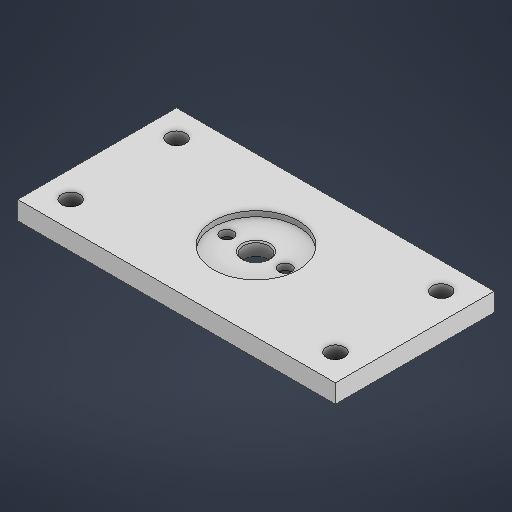
# Autodesk Inventor part: motor mount plate
Saved by Autodesk Inventor 2025.2 (Build 292293000, 293)
## iProperties
Created: 2025-05-10
Part Number: motor mount plate
Material: Generic
Document SubType Name: Modeling
Designer: klawy
Density: 1 g/cm^3
Appearance: Default
Author: klawy
Autodesk Inventor part; units mm, degrees
ref_plane "YZ Plane" through (0, 0, 0) normal (1, 0, 0) x (0, 1, 0)
ref_plane "XZ Plane" through (0, 0, 0) normal (0, 1, 0) x (-1, 0, 0)
ref_plane "XY Plane" through (0, 0, 0) normal (0, 0, 1) x (1, 0, 0)
sketch "Sketch1" plane through (0, 0, 0) normal (0, 1, 0) x (-1, 0, 0)
  circle A0 centre (0, 0) radius 8 construction
  circle A1 centre (0, 0) radius 2.35
  line L0 (30, 15) -> (-30, 15)
  line L1 (-30, 15) -> (-30, -15)
  line L2 (-30, -15) -> (30, -15)
  line L3 (30, -15) -> (30, 15)
  line L4 (0, -21) -> (0, 21) projected
  point P0 (0, 15)
  dimension "d0" = 16
  dimension "d3" = 4.7
  dimension "d4" = 60
  dimension "d5" = 30
  dimension "d6" = 15
  constraints: 8 end point, 2 centre point, 2 coincident, 2 parallel, 1 horizontal, 1 midpoint, 1 perpendicular, 1 point on line
  measures "d0" diameter of A0
  measures "d3" diameter of A1
  measures "d4" distance of L0.start L0.end
  measures "d5" distance of L0.end L1.end
  measures "d6" distance from line of L0 point (0, 0)
extrude "Extrusion1" add sketch "Sketch1" along normal blind 2.5 contours A1 L4 L0 L3 L2 | A1 L4 L2 L1 L0
sketch "Sketch2" plane through (0, 2.5, 0) normal (0, 1, 0) x (1, 0, 0)
  circle A0 centre (0, 0) radius 3.5
  line L0 (-30, 15) -> (-30, -15) projected
  line L1 (-30, -15) -> (30, -15) projected
  line L2 (30, -15) -> (30, 15) projected
  line L3 (30, 15) -> (-30, 15) projected
  circle A1 centre (0, 0) radius 2.35 projected
  dimension "d9" = 7
  constraints: 1 centre point, 1 coincident
  measures "d9" diameter of A0
extrude "Extrusion2" add sketch "Sketch2" along normal blind 1 contours L3 L2 L1 L0
sketch "Sketch4" plane through (0, 0, 0) normal (0, -1, 0) x (1, 0, 0)
  line L0 (-42, 0) -> (42, 0) projected
  point P0 (0, 0)
  point P1 (-5.5, 0)
  point P2 (5.5, 0)
  dimension "d18" = 360
  dimension "d20" = 5.5
  constraints: 1 point on line, 3 other
  measures "d20" distance of point (0, 0) point (-5.5, 0)
hole "Hole1" at (-5.5, 0, 0) at (5.5, 0, 0) direction (0, 1, 0) diameter 2.4 end through all counterbore diameter 4.4 counterbore depth 2.3 clearance for "Socket Head Cap Screw ISO 4762" size "M2" standard "ISO"
sketch "Sketch5" plane through (0, 2.5, 0) normal (0, 1, 0) x (1, 0, 0)
  circle A0 centre (0, 0) radius 8
  dimension "d30" = 16
  constraints: 1 centre point, 1 coincident
  measures "d30" diameter of A0
extrude "Extrusion3" cut sketch "Sketch5" along normal blind 1
sketch "Sketch7" plane through (0, 0, 0) normal (0, -1, 0) x (1, 0, 0)
  circle A0 centre (-25, 10) radius 4
  line L0 (-30, 15) -> (30, 15) projected
  line L1 (-30, -15) -> (-30, 15) projected
  circle A1 centre (25, 10) radius 4
  circle A2 centre (-25, -10) radius 4
  circle A3 centre (25, -10) radius 4
  point P0 (0, 0)
  dimension "d34" = 8
  dimension "d35" = 5
  dimension "d36" = 5
  dimension "d39" = 50
  dimension "d42" = 20
  constraints: 4 centre point, 1 horizontal, 1 vertical, 6 other
  measures "d34" diameter of A0
  measures "d35" distance from line of L0 A0.centre
  measures "d36" distance from line of L1 A0.centre
  measures "d39" distance of A0.centre A1.centre
  measures "d42" distance of A0.centre A2.centre
extrude "Extrusion4" cut sketch "Sketch7" against normal blind 1
chamfer "Chamfer1" distance 0.25 angle 45 1 edges at (2.35, 2.5, 0)
sketch "Sketch9" plane through (0, 3.5, 0) normal (0, 1, 0) x (1, 0, 0)
  circle A0 centre (-25, -10) radius 4 construction
  point P0 (0, 0)
  constraints: 1 coincident
hole "Hole2" at (-25, 3.5, 10) direction (0, -1, 0) diameter 3.4 end through all clearance for "Socket Head Cap Screw ISO 4762" size "M3" standard "ISO"
pattern_linear "Rectangular Pattern1" count 2 spacing 20 along (0, 0, -1) count 2 spacing 50 along (1, 0, 0) of "Hole2"
sketch "Sketch10" plane through (5.5, 2.3, 0) normal (0, -1, 0) x (1, 0, 0)
  circle A0 centre (0, 0) radius 2.2 projected
  circle A1 centre (0, 0) radius 1.2 projected
  circle A2 centre (-11, 0) radius 2.2 projected
  circle A3 centre (-11, 0) radius 1.2 projected
  point P0 (-5.5, 0)
extrude "Extrusion6" add sketch "Sketch10" along normal blind 1
body "Solid1"
